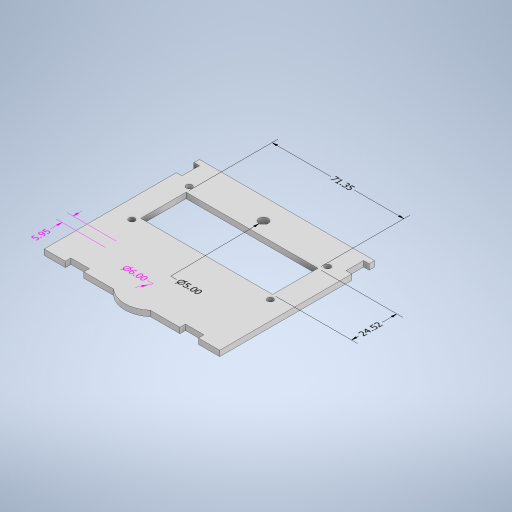
# Autodesk Inventor part: Tampa
Saved by Autodesk Inventor 2024 (Build 280153000, 153)
## iProperties
Created: 2023-11-29
Part Number: Tampa
Material: Genérico
Document SubType Name: Modeling
Designer: caiot
Density: 1 g/cm^3
Appearance: Padrão
Author: caiot
Autodesk Inventor part; units mm, degrees
ref_plane "YZ Plane" through (0, 0, 0) normal (1, 0, 0) x (0, 1, 0)
ref_plane "XZ Plane" through (0, 0, 0) normal (0, 1, 0) x (-1, 0, 0)
ref_plane "XY Plane" through (0, 0, 0) normal (0, 0, 1) x (1, 0, 0)
sketch "Esboço3" plane through (0, 0, 0) normal (0, 1, 0) x (-1, 0, 0)
  line L0 (0, 0) -> (-95, 0)
  line L1 (-95, 0) -> (-95, -80)
  line L2 (-95, -80) -> (0, -80)
  line L3 (0, -80) -> (0, 0)
  line L4 (-11.825, -65) -> (-83.175, -65)
  line L5 (-83.175, -65) -> (-83.175, -40.48)
  line L6 (-83.175, -40.48) -> (-11.825, -40.48)
  line L7 (-11.825, -40.48) -> (-11.825, -65)
  circle A0 centre (-46.25, -72.5) radius 2.5
  point P0 (-47.5, -40.48)
  dimension "d4" = 95
  dimension "d5" = 80
  dimension "d9" = 71.35
  dimension "d10" = 24.52
  dimension "d11" = 11.825
  dimension "d17" = 5
  dimension "d56" = 15
  dimension "d140" = 11.825
  dimension "d251" = 40.48
  dimension "d259" = 7.5
  constraints: 16 end point, 4 parallel, 2 horizontal, 2 perpendicular, 1 centre point, 1 midpoint
  measures "d4" distance of L2.end L1.end
  measures "d5" distance of L1.end L0.end
  measures "d9" distance of L5.end L6.end
  measures "d10" distance of L4.end L5.end
  measures "d11" distance between parallel lines of L3 L7
  measures "d17" diameter of A0
  measures "d56" distance between parallel lines of L2 L4
  measures "d140" distance between parallel lines of L1 L5
  measures "d251" distance between parallel lines of L0 L6
  measures "d259" distance from line of A0.centre L2
extrude "Extrusão2" add sketch "Esboço3" along normal blind 3
sketch "Esboço7" plane through (0, 3, 0) normal (0, 1, 0) x (1, 0, 0)
  line L0 (10, 68.48) -> (85, 68.48)
  line L1 (85, 68.48) -> (85, 37.48)
  line L2 (85, 37.48) -> (10, 37.48)
  line L3 (10, 37.48) -> (10, 68.48)
  line L4 (11.825, 40.48) -> (11.825, 65) projected
  line L5 (83.175, 65) -> (83.175, 40.48) projected
  line L6 (11.825, 65) -> (83.175, 65) projected
  line L7 (83.175, 40.48) -> (11.825, 40.48) projected
  circle A0 centre (10, 37.48) radius 1.6
  circle A1 centre (10, 68.48) radius 1.6
  circle A2 centre (85, 68.48) radius 1.6
  circle A3 centre (85, 37.48) radius 1.6
  point P0 (0, 0)
  dimension "d57" = 75
  dimension "d58" = 31
  dimension "d59" = 1.825
  dimension "d60" = 73.175
  dimension "d62" = 1.825
  dimension "d65" = 3.2
  dimension "d66" = 3.2
  dimension "d67" = 3.2
  dimension "d68" = 3.2
  dimension "d69" = 3
  constraints: 8 end point, 4 centre point, 4 coincident, 2 parallel, 1 horizontal, 1 perpendicular
  measures "d57" distance of L1.end L2.end
  measures "d58" distance of L0.end L1.end
  measures "d59" distance between parallel lines of L4 L3
  measures "d60" distance between parallel lines of L1 L4
  measures "d62" distance between parallel lines of L5 L1
  measures "d65" diameter of A0
  measures "d66" diameter of A1
  measures "d67" diameter of A2
  measures "d68" diameter of A3
  measures "d69" distance between parallel lines of L2 L7
extrude "Extrusão4" cut sketch "Esboço7" against normal blind 3 contours L3 A1 L0 | L0 A1 L3 | A2 L1 L0 | L0 L1 A2 | A0 L2 L3 | L3 L2 A0 | A3 L2 L1 | L1 L2 A3
sketch "Esboço19" plane through (0, 3, 0) normal (0, 1, 0) x (1, 0, 0)
  line L0 (0, 0) -> (95, 0) projected
  arc A0 (37.5, 0) -> (57.5, 0) centre (47.5, 11.1803) ccw
  dimension "d189" = 20
  dimension "d190" = 15
  dimension "d191" = 37.5
  constraints: 2 point on circle, 2 point on line, 1 centre point
  measures "d189" distance of A0.start A0.end
  measures "d190" radius of A0
  measures "d191" distance of L0.start A0.start
extrude "Extrusão14" add sketch "Esboço19" against normal blind 3
sketch "Esboço23" plane through (0, 3, 0) normal (0, 1, 0) x (1, 0, 0)
  line L0 (0, 80) -> (0, 0) projected
  line L1 (0, 80) -> (95, 80)
  line L2 (95, 80) -> (95, 84)
  line L3 (95, 84) -> (0, 84)
  line L4 (0, 84) -> (0, 80)
  dimension "d208" = 4
  constraints: 8 end point, 2 parallel, 1 horizontal, 1 perpendicular
  measures "d208" distance of L2.end L1.end
extrude "Extrusão17" add sketch "Esboço23" against normal blind 3
sketch "Esboço24" plane through (0, 3, 0) normal (0, 1, 0) x (1, 0, 0)
  line L0 (95, 0) -> (95, 84) projected
  line L1 (95, 71.5) -> (91.9, 71.5)
  line L2 (91.9, 71.5) -> (91.9, 84)
  line L3 (91.9, 84) -> (95, 84)
  line L4 (95, 84) -> (95, 71.5)
  line L5 (95, 84) -> (0, 84) projected
  point P0 (0, 0)
  point P1 (93.45, 84)
  dimension "d211" = 3.1
  dimension "d212" = 12.5
  dimension "d213" = 0
  constraints: 8 end point, 2 parallel, 1 horizontal, 1 midpoint, 1 perpendicular, 1 point on line
  measures "d211" distance of L2.end L3.end
  measures "d212" distance of L1.end L2.end
  measures "d213" distance from line of L5 point (93.45, 84)
extrude "Extrusão18" cut sketch "Esboço24" against normal blind 3
sketch "Esboço27" plane through (0, 3, 0) normal (0, 1, 0) x (1, 0, 0)
  line L0 (91.9, 84) -> (0, 84) projected
  line L1 (0, 84) -> (3, 84)
  line L2 (3, 84) -> (3, 71.5)
  line L3 (3, 71.5) -> (0, 71.5)
  line L4 (0, 71.5) -> (0, 84)
  point P0 (0, 0)
  dimension "d226" = 3
  dimension "d227" = 12.5
  constraints: 8 end point, 2 parallel, 1 horizontal, 1 perpendicular
  measures "d226" distance of L2.end L3.end
  measures "d227" distance of L1.end L2.end
extrude "Extrusão21" cut sketch "Esboço27" against normal blind 3
sketch "Esboço29" plane through (0, 3, 0) normal (0, 1, 0) x (1, 0, 0)
  line L0 (57.5, 0) -> (95, 0) projected
  line L1 (83.5, 0) -> (73.5, 0)
  line L2 (73.5, 0) -> (73.5, 3)
  line L3 (73.5, 3) -> (83.5, 3)
  line L4 (83.5, 3) -> (83.5, 0)
  line L5 (21.5, 0) -> (11.5, 0)
  line L6 (11.5, 0) -> (11.5, 3)
  line L7 (11.5, 3) -> (21.5, 3)
  line L8 (21.5, 3) -> (21.5, 0)
  line L9 (0, 71.5) -> (0, 0) projected
  line L10 (95, 0) -> (95, 71.5) projected
  point P0 (11.5, 1.5)
  point P1 (83.5, 1.5)
  dimension "d241" = 10
  dimension "d242" = 3
  dimension "d243" = 10
  dimension "d244" = 3
  dimension "d245" = 11.5
  dimension "d246" = 11.5
  constraints: 16 end point, 4 parallel, 2 horizontal, 2 midpoint, 2 perpendicular, 2 point on line
  measures "d241" distance of L2.end L3.end
  measures "d242" distance of L1.end L2.end
  measures "d243" distance of L6.end L7.end
  measures "d244" distance of L5.end L6.end
  measures "d245" distance from line of L9 point (11.5, 1.5)
  measures "d246" distance from line of L10 point (83.5, 1.5)
extrude "Extrusão23" cut sketch "Esboço29" against normal blind 3
sketch "Esboço30" plane through (0, 3, 0) normal (0, 1, 0) x (1, 0, 0)
  line L0 (91.9, 71.5) -> (91.9, 84) projected
  line L1 (91.9, 84) -> (94.9, 84)
  line L2 (94.9, 84) -> (94.9, 81)
  line L3 (94.9, 81) -> (91.9, 81)
  line L4 (91.9, 81) -> (91.9, 84)
  line L5 (3, 71.5) -> (3, 84) projected
  line L6 (3, 84) -> (0, 84)
  line L7 (0, 84) -> (0, 81)
  line L8 (0, 81) -> (3, 81)
  line L9 (3, 81) -> (3, 84)
  point P0 (0, 0)
  dimension "d253" = 3
  dimension "d254" = 3
  dimension "d255" = 3
  dimension "d256" = 3
  constraints: 16 end point, 4 parallel, 2 horizontal, 2 perpendicular
  measures "d253" distance of L2.end L3.end
  measures "d254" distance of L1.end L2.end
  measures "d255" distance of L8.end L7.end
  measures "d256" distance of L7.end L6.end
extrude "Extrusão24" add sketch "Esboço30" against normal blind 3
